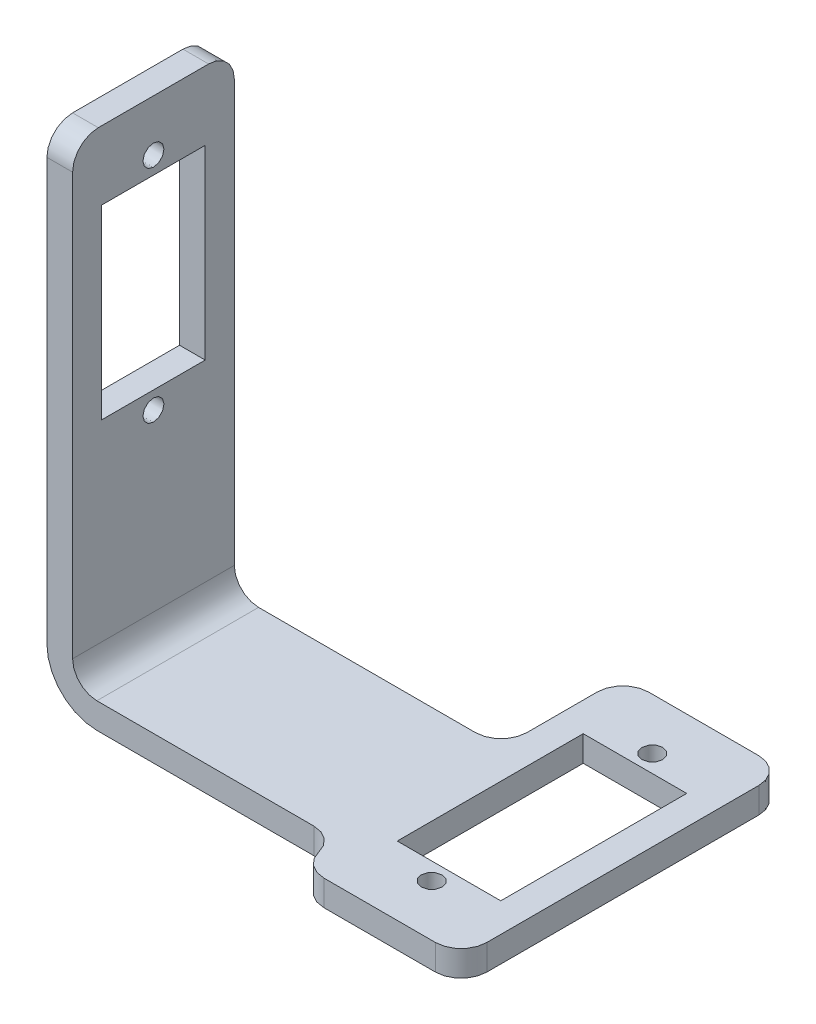
# Autodesk Inventor part: Midplate
Saved by Autodesk Inventor 2023.4 (Build 274418000, 418)
## iProperties
Created: 2024-05-24
Part Number: Midplate
Material: Generic
Document SubType Name: Modeling
Designer: Nathan Cai
Density: 1 g/cm^3
Appearance: Rubber - Black
Author: Nathan Cai
Autodesk Inventor part; units mm, degrees
ref_plane "YZ Plane" through (0, 0, 0) normal (1, 0, 0) x (0, 1, 0)
ref_plane "XZ Plane" through (0, 0, 0) normal (0, 1, 0) x (-1, 0, 0)
ref_plane "XY Plane" through (0, 0, 0) normal (0, 0, 1) x (1, 0, 0)
sketch "Sketch2" plane through (0, 0, 0) normal (0, 1, 0) x (-1, 0, 0)
  line L0 (-6.4, 11.5) -> (6.4, 11.5)
  line L1 (6.4, 11.5) -> (6.4, -11.5)
  line L2 (6.4, -11.5) -> (-6.4, -11.5)
  line L3 (-6.4, -11.5) -> (-6.4, 11.5)
  line L4 (-6.4, 11.5) -> (6.4, -11.5) construction
  line L5 (6.4, 11.5) -> (-6.4, -11.5) construction
  circle A0 centre (0, 0) radius 13.65 construction
  line L6 (0, 0) -> (0, -13.65) construction
  circle A1 centre (0, -13.65) radius 1.3
  circle A2 centre (0, 13.65) radius 1.3
  line L7 (-10, 20) -> (10, 20)
  line L8 (10, 20) -> (10, -20)
  line L9 (10, -20) -> (-10, -20)
  line L10 (-10, -20) -> (-10, 20)
  line L11 (-10, 20) -> (10, -20) construction
  line L12 (10, 20) -> (-10, -20) construction
  line L13 (-10, 5.05) -> (10, 5.05) construction
  line L14 (10, 15.05) -> (100, 15.05)
  line L15 (100, 15.05) -> (100, -4.95)
  line L16 (100, -4.95) -> (10, -4.95)
  line L17 (10, -4.95) -> (10, 15.05)
  line L18 (100, 5.05) -> (10, 5.05) construction
  line L19 (91.5, 11.45) -> (68.5, 11.45)
  line L20 (68.5, 11.45) -> (68.5, -1.35)
  line L21 (68.5, -1.35) -> (91.5, -1.35)
  line L22 (91.5, -1.35) -> (91.5, 11.45)
  line L23 (91.5, 11.45) -> (68.5, -1.35) construction
  line L24 (68.5, 11.45) -> (91.5, -1.35) construction
  circle A3 centre (80, 5.05) radius 13.65 construction
  circle A4 centre (93.65, 5.05) radius 1.3
  circle A5 centre (66.35, 5.05) radius 1.3
  dimension "d2" = 27.3
  dimension "d20" = 27.3
  dimension "d0" = 12.8
  dimension "d1" = 23
  dimension "d3" = 2.6
  dimension "d6" = 360
  dimension "d8" = 20
  dimension "d9" = 40
  dimension "d11" = 8.6
  dimension "d12" = 90
  dimension "d14" = 20
  dimension "d18" = 12.8
  dimension "d19" = 23
  dimension "d21" = 2.6
  dimension "d24" = 360
  dimension "d26" = 20
  constraints: 50 end point, 8 parallel, 7 midpoint, 6 perpendicular, 6 point on line, 4 centre point, 4 horizontal, 3 coincident, 1 horizontal alignment, 1 vertical, 1 vertical alignment, 14 other
  measures "d0" distance of L1.end L2.end
  measures "d1" distance of L0.end L1.end
  measures "d3" diameter of A1
  measures "d8" distance of L8.end L9.end
  measures "d9" distance of L7.end L8.end
  measures "d11" distance from line of L13 A2.centre
  measures "d12" distance of L15.end L16.end
  measures "d14" distance between parallel lines of L14 L16
  measures "d18" distance between parallel lines of L19 L21
  measures "d19" distance between parallel lines of L20 L22
  measures "d21" diameter of A4
  measures "d26" distance from line of L15 point (80, 5.05)
extrude "Extrusion1" add sketch "Sketch2" along normal blind 3.175
fillet "Fillet1" radius 3.175 8 edges at (-10, 1.5875, 15.05) (-10, 1.5875, 20) (10, 1.5875, 20) (10, 1.5875, -20) (-10, 1.5875, -20) (-10, 1.5875, -4.95) (-100, 1.5875, -4.95) (-100, 1.5875, 15.05)
sketch "Sketch3" plane through (0, 3.175, 0) normal (0, 1, 0) x (1, 0, 0)
  line L0 (-96.825, -15.05) -> (-13.175, -15.05) projected
  line L1 (-40, -15.05) -> (-40, 4.95)
  line L2 (-13.175, 4.95) -> (-96.825, 4.95) projected
  line L3 (10, -16.825) -> (10, 16.825) projected
  point P0 (0, 0)
  dimension "d27" = 50
  constraints: 2 end point, 2 point on line, 1 vertical
  measures "d27" distance between parallel lines of L3 L1
bend part "Bend Part1" radius 3 angle 90 line through (-40, 3.175, 15.05) along (0, 0, -1) centre toward (0, 1, 0) moving side (-1, 0, 0) both sides no
equation "\"d20\" = d2"
equation "\"d18\" = d0"
equation "\"d19\" = d1"
equation "\"d21\" = d3"
body "Solid1"
